Autodesk Fusion 360 part; units mm, degrees
(part 2 of 2)
sketch "Sketch2" plane through (77.4, 0, 0) normal (1, 0, 0) x (0, 1, 0)
  line L0 (0, 36.6134) -> (0, 2)
  line L1 (0, 2) -> (150, 2)
  line L2 (150, 2) -> (150, 36.6134)
  line L3 (150, 36.6134) -> (0, 36.6134)
  line L4 (0, 44) -> (0, 2)
  line L5 (150, 44) -> (0, 44)
  line L6 (150, 11) -> (0, 11)
  line L7 (150, 7) -> (0, 7)
  line L8 (150, 2) -> (150, 44)
  line L9 (0, 2) -> (150, 2)
  line L10 (150, 36) -> (0, 36)
  line L11 (0, 37) -> (150, 37)
  line L12 (150, 29) -> (150, 28)
  line L13 (0, 10) -> (150, 10)
  line L14 (0, 9) -> (0, 10)
  line L15 (150, 38) -> (0, 38)
  line L16 (150, 8) -> (150, 7)
  line L17 (0, 32) -> (0, 33)
  line L18 (150, 35) -> (150, 34)
  line L19 (150, 30) -> (0, 30)
  line L20 (0, 39) -> (150, 39)
  line L21 (150, 9) -> (0, 9)
  line L22 (0, 6) -> (150, 6)
  line L23 (0, 38) -> (0, 39)
  line L24 (0, 28) -> (0, 29)
  line L25 (0, 36) -> (0, 37)
  line L26 (0, 11) -> (0, 12)
  line L27 (0, 29) -> (150, 29)
  line L28 (150, 12) -> (150, 11)
  line L29 (0, 31) -> (150, 31)
  line L30 (150, 5) -> (0, 5)
  line L31 (0, 33) -> (150, 33)
  line L32 (150, 31) -> (150, 30)
  line L33 (0, 35) -> (150, 35)
  line L34 (150, 6) -> (150, 5)
  line L35 (150, 10) -> (150, 9)
  line L36 (150, 28) -> (0, 28)
  line L37 (0, 12) -> (150, 12)
  line L38 (0, 8) -> (150, 8)
  line L39 (150, 37) -> (150, 36)
  line L40 (0, 7) -> (0, 8)
  line L41 (0, 30) -> (0, 31)
  line L42 (0, 34) -> (0, 35)
  line L43 (150, 32) -> (0, 32)
  line L44 (0, 5) -> (0, 6)
  line L45 (150, 39) -> (150, 38)
  line L46 (150, 33) -> (150, 32)
  line L47 (150, 34) -> (0, 34)
  point P0 (150, 0)
  dimension "d78" = 150
  dimension "d79" = 1
  dimension "d80" = 150
  dimension "d81" = 1
  dimension "d82" = 150
  dimension "d83" = 1
  dimension "d84" = 150
  dimension "d85" = 1
  dimension "d86" = 150
  dimension "d87" = 1
  dimension "d88" = 150
  dimension "d89" = 1
  dimension "d90" = 1
  dimension "d91" = 1
  dimension "d92" = 1
  dimension "d93" = 1
  dimension "d94" = 1
  dimension "d96" = 5
  dimension "d97" = 150
  dimension "d98" = 1
  dimension "d99" = 150
  dimension "d100" = 1
  dimension "d101" = 150
  dimension "d102" = 1
  dimension "d103" = 150
  dimension "d104" = 1
  dimension "d105" = 1
  dimension "d106" = 1
  dimension "d107" = 1
  dimension "d108" = 3
  constraint horizontal L20
  constraint vertical L45
  constraint horizontal L15
  constraint vertical L23
  constraint coincident L20.start L4
  constraint horizontal L11
  constraint vertical L39
  constraint horizontal L10
  constraint vertical L25
  constraint coincident L11.start L4
  constraint horizontal L33
  constraint vertical L18
  constraint horizontal L47
  constraint vertical L42
  constraint coincident L33.start L4
  constraint horizontal L29
  constraint vertical L32
  constraint horizontal L19
  constraint vertical L41
  constraint horizontal L31
  constraint vertical L46
  constraint horizontal L43
  constraint vertical L17
  constraint coincident L17.end L4
  constraint horizontal L27
  constraint vertical L12
  constraint horizontal L36
  constraint vertical L24
  constraint coincident L24.end L4
  constraint horizontal L13
  constraint vertical L35
  constraint horizontal L21
  constraint vertical L14
  constraint coincident L13.start L4
  constraint horizontal L38
  constraint vertical L16
  constraint horizontal L7
  constraint vertical L40
  constraint coincident L38.start L4
  constraint horizontal L22
  constraint vertical L34
  constraint horizontal L30
  constraint vertical L44
  constraint coincident L22.start L4
  constraint horizontal L37
  constraint vertical L28
  constraint horizontal L6
  constraint vertical L26
  constraint coincident L26.end L4
  measures "d78" distance of L20.start L20.end
  measures "d79" distance of L20.start L15.end
  measures "d80" distance of L11.end L11.start
  measures "d81" distance of L10.end L11.start
  measures "d82" distance of L33.start L18.start
  measures "d83" distance of L42.start L33.start
  measures "d84" distance of L29.end L29.start
  measures "d85" distance of L19.end L29.start
  measures "d86" distance of L17.end L31.end
  measures "d87" distance of L17.start L17.end
  measures "d88" distance of L12.start L24.end
  measures "d89" distance of L24.start L24.end
  measures "d90" distance of L11 L15
  measures "d91" distance of L10 L33
  measures "d92" distance of L31 L47
  measures "d93" distance of L19 L27
  measures "d94" distance of L29 L43
  measures "d96" distance of L5 L20
  measures "d97" distance of L13.start L13.end
  measures "d98" distance of L13.start L14.start
  measures "d99" distance of L38.start L16.start
  measures "d100" distance of L38.start L7.end
  measures "d101" distance of L22.start L22.end
  measures "d102" distance of L30.end L22.start
  measures "d103" distance of L26.end L28.start
  measures "d104" distance of L26.end L6.end
  measures "d105" distance of L7 L22
  measures "d106" distance of L21 L38
  measures "d107" distance of L6 L13
  measures "d108" distance of L9 L30
extrude "Extrude2" cut sketch "Sketch2" against normal blind 1 contours L0 L2 L4 L8 L18 L33 L42 L47 | L0 L2 L4 L8 L17 L31 L43 L46 | L0 L2 L4 L8 L19 L29 L32 L41 | L0 L2 L4 L8 L12 L24 L27 L36 | L0 L2 L4 L6 L8 L26 L28 L37 | L0 L2 L4 L8 L13 L14 L21 L35 | L0 L2 L4 L7 L8 L16 L38 L40 | L0 L2 L4 L8 L22 L30 L34 L44
sketch "Sketch3" plane through (0, 0, 0) normal (-1, 0, 0) x (0, -1, 0)
  line L0 (0, 2) -> (0, 36.6134)
  line L1 (0, 36.6134) -> (-150, 36.6134)
  line L2 (-150, 36.6134) -> (-150, 2)
  line L3 (-150, 2) -> (0, 2)
  line L4 (-150, 10) -> (-150, 11)
  line L5 (-150, 33) -> (-150, 34)
  line L6 (0, 4) -> (0, 5)
  line L7 (0, 6) -> (0, 7)
  line L8 (0, 8) -> (0, 9)
  line L9 (0, 11) -> (0, 10)
  line L10 (-150, 44) -> (-150, 2)
  line L11 (-150, 30) -> (0, 30)
  line L12 (0, 28) -> (0, 27)
  line L13 (-150, 38) -> (0, 38)
  line L14 (0, 29) -> (-150, 29)
  line L15 (-150, 7) -> (-150, 6)
  line L16 (0, 5) -> (-150, 5)
  line L17 (-150, 34) -> (0, 34)
  line L18 (-150, 37) -> (-150, 38)
  line L19 (-150, 4) -> (0, 4)
  line L20 (0, 37) -> (-150, 37)
  line L21 (-150, 8) -> (0, 8)
  line L22 (0, 33) -> (-150, 33)
  line L23 (-150, 6) -> (0, 6)
  line L24 (0, 7) -> (-150, 7)
  line L25 (-150, 5) -> (-150, 4)
  line L26 (0, 10) -> (-150, 10)
  line L27 (0, 9) -> (-150, 9)
  line L28 (-150, 27) -> (-150, 28)
  line L29 (-150, 11) -> (0, 11)
  line L30 (-150, 29) -> (-150, 30)
  line L31 (-150, 9) -> (-150, 8)
  line L32 (0, 27) -> (-150, 27)
  line L33 (-150, 28) -> (0, 28)
  line L34 (0, 34) -> (0, 33)
  line L35 (0, 31) -> (-150, 31)
  line L36 (0, 32) -> (0, 31)
  line L37 (0, 36) -> (0, 35)
  line L38 (-150, 32) -> (0, 32)
  line L39 (-150, 36) -> (0, 36)
  line L40 (0, 2) -> (0, 44)
  line L41 (0, 44) -> (-150, 44)
  line L42 (-150, 2) -> (0, 2)
  line L43 (0, 38) -> (0, 37)
  line L44 (-150, 31) -> (-150, 32)
  line L45 (-150, 35) -> (-150, 36)
  line L46 (0, 30) -> (0, 29)
  line L47 (0, 35) -> (-150, 35)
  point P0 (-150, 0)
  dimension "d111" = 150
  dimension "d112" = 1
  dimension "d113" = 150
  dimension "d114" = 1
  dimension "d115" = 150
  dimension "d116" = 1
  dimension "d117" = 150
  dimension "d118" = 1
  dimension "d119" = 150
  dimension "d120" = 1
  dimension "d121" = 150
  dimension "d122" = 1
  dimension "d123" = 150
  dimension "d124" = 1
  dimension "d125" = 150
  dimension "d126" = 1
  dimension "d127" = 150
  dimension "d128" = 1
  dimension "d129" = 150
  dimension "d130" = 1
  constraint horizontal L13
  constraint vertical L43
  constraint horizontal L20
  constraint vertical L18
  constraint coincident L13.start L10
  constraint horizontal L39
  constraint vertical L37
  constraint horizontal L47
  constraint vertical L45
  constraint coincident L39.start L10
  constraint horizontal L17
  constraint vertical L34
  constraint horizontal L22
  constraint vertical L5
  constraint coincident L5.end L10
  constraint horizontal L38
  constraint vertical L36
  constraint horizontal L35
  constraint vertical L44
  constraint coincident L38.start L10
  constraint horizontal L11
  constraint vertical L46
  constraint horizontal L14
  constraint vertical L30
  constraint coincident L11.start L10
  constraint horizontal L33
  constraint vertical L12
  constraint horizontal L32
  constraint vertical L28
  constraint coincident L28.end L10
  constraint horizontal L19
  constraint vertical L6
  constraint horizontal L16
  constraint vertical L25
  constraint coincident L19.start L10
  constraint horizontal L23
  constraint vertical L7
  constraint horizontal L24
  constraint vertical L15
  constraint coincident L15.end L10
  constraint horizontal L21
  constraint vertical L8
  constraint horizontal L27
  constraint vertical L31
  constraint coincident L21.start L10
  constraint horizontal L29
  constraint vertical L9
  constraint horizontal L26
  constraint vertical L4
  constraint coincident L4.end L10
  measures "d111" distance of L13.end L13.start
  measures "d112" distance of L18.start L13.start
  measures "d113" distance of L37.start L39.start
  measures "d114" distance of L39.start L45.start
  measures "d115" distance of L17.end L5.end
  measures "d116" distance of L5.start L5.end
  measures "d117" distance of L38.start L36.start
  measures "d118" distance of L35.end L38.start
  measures "d119" distance of L11.start L11.end
  measures "d120" distance of L11.start L14.end
  measures "d121" distance of L28.end L12.start
  measures "d122" distance of L28.end L28.start
  measures "d123" distance of L19.start L6.start
  measures "d124" distance of L16.end L19.start
  measures "d125" distance of L15.end L7.start
  measures "d126" distance of L15.start L15.end
  measures "d127" distance of L8.start L21.start
  measures "d128" distance of L21.start L27.end
  measures "d129" distance of L4.end L9.start
  measures "d130" distance of L4.end L4.start
extrude "Extrude3" cut sketch "Sketch3" against normal blind 1 contours L0 L2 L6 L10 L16 L19 L25 L40 | L0 L2 L7 L10 L15 L23 L24 L40 | L0 L2 L8 L10 L21 L27 L31 L40 | L0 L2 L4 L9 L10 L26 L29 L40 | L0 L2 L10 L12 L28 L32 L33 L40 | L0 L2 L10 L11 L14 L30 L40 L46 | L0 L2 L10 L35 L36 L38 L40 L44 | L0 L2 L5 L10 L17 L22 L34 L40 | L0 L2 L10 L37 L39 L40 L45 L47

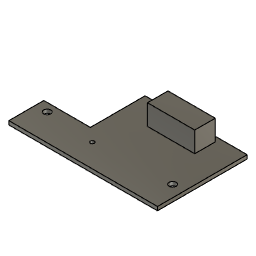
design "InputBoard"
Autodesk Fusion 360 part; units mm, degrees
sketch "Sketch1" plane through (0, 0, 0) normal (0, 0, 1) x (1, 0, 0)
  line L0 (0, 0) -> (63.8, 0)
  line L1 (63.8, 0) -> (63.8, 38.5)
  line L2 (63.8, 38.5) -> (0, 38.5)
  line L3 (0, 38.5) -> (0, 0)
  line L4 (0, 15) -> (20, 15)
  line L5 (20, 15) -> (20, 38.5)
  line L6 (63.8, 38.5) -> (43.8, 38.5)
  line L7 (43.8, 38.5) -> (52.6, 38.5)
  line L8 (52.6, 38.5) -> (52.6, 0)
  line L9 (52.6, 0) -> (43.8, 0)
  line L10 (43.8, 0) -> (43.8, 38.5)
  dimension "d1" = 63.8
  dimension "d2" = 38.5
  dimension "d3" = 20
  dimension "d4" = 15
  dimension "d5" = 20
  dimension "d6" = 8.8
  dimension "d7" = 38.5
  constraint horizontal L0
  constraint vertical L1
  constraint horizontal L2
  constraint vertical L3
  constraint coincident L0.start L3.end
  constraint coincident L3 L4.start
  constraint perpendicular L3 L4
  constraint coincident L2 L5.end
  constraint perpendicular L2 L5
  constraint perpendicular L1 L6
  constraint horizontal L7
  constraint vertical L8
  constraint horizontal L9
  constraint vertical L10
  measures "d1" distance of L0.start L0.end
  measures "d2" distance of L0.start L2.end
  measures "d3" distance of L4.start L4.end
  measures "d4" distance of L0 L4
  measures "d5" distance of L1.end L6.end
  measures "d6" distance of L6.end L7.end
  measures "d7" distance of L6.end L9.end
extrude "Extrude2" add sketch "Sketch1" along normal blind 1.6 contours L0 L2 L3 L4 L5 L10 | L0 L2 L6 L7 L8 L9 L10 | L0 L1 L2 L6 L8
sketch "Sketch4" plane through (0, 0, 1.6) normal (0, 0, 1) x (-1, 0, 0)
  line L0 (-63.8, 0) -> (-63.8, -38.5)
  line L1 (-63.8, -38.5) -> (-20, -38.5)
  line L2 (-20, -38.5) -> (-20, -15)
  line L3 (-20, -15) -> (0, -15)
  line L4 (0, -15) -> (0, 0)
  line L5 (0, 0) -> (-63.8, 0)
  circle A0 centre (-5, -11.5) radius 1.5
  circle A1 centre (-58.8, -11.5) radius 1.5
  dimension "d23" = 3
  dimension "d24" = 11.5
  dimension "d25" = 5
  dimension "d28" = 3
  dimension "d39" = 58.8
  constraint horizontal A0.centre A1.centre
  measures "d23" diameter of A0
  measures "d24" distance of L5 A0.centre
  measures "d25" distance of L4 A0.centre
  measures "d28" diameter of A1
  measures "d39" distance of L4 A1.centre
extrude "Extrude5" cut sketch "Sketch4" against normal blind 1.6 contours A0
hole "Hole1" at (58.8, 11.5, 1.6) direction (0, 0, -1) diameter 3 depth 5 tip angle 180
sketch "Sketch5" plane through (0, 0, 1.6) normal (0, 0, 1) x (1, 0, 0)
  circle A0 centre (25.907, 9.929) radius 0.85
  line L0 (0, 0) -> (63.8, 0)
  line L1 (0, 15) -> (0, 0)
  dimension "d34" = 1.7
  dimension "d35" = 9.929
  dimension "d36" = 25.907
  measures "d34" diameter of A0
  measures "d35" distance of A0.centre L0
  measures "d36" distance of A0.centre L1
extrude "Extrude6" cut sketch "Sketch5" against normal blind 1.6
sketch "Sketch6" plane through (0, 0, 1.6) normal (0, 0, 1) x (-1, 0, 0)
  circle A0 centre (-25.907, -9.929) radius 0.85
  circle A1 centre (-58.8, -11.5) radius 1.5
  circle A2 centre (-5, -11.5) radius 1.5
  line L0 (-63.8, 0) -> (-63.8, -38.5)
  line L1 (-63.8, -38.5) -> (-20, -38.5)
  line L2 (-20, -38.5) -> (-20, -15)
  line L3 (-20, -15) -> (0, -15)
  line L4 (0, -15) -> (0, 0)
  line L5 (0, 0) -> (-63.8, 0)
  line L6 (-52.187, -27.604) -> (-31.887, -27.604)
  line L7 (-31.887, -27.604) -> (-31.887, -36.404)
  line L8 (-31.887, -36.404) -> (-52.187, -36.404)
  line L9 (-52.187, -36.404) -> (-52.187, -27.604)
  line L10 (-52.187, -27.604) -> (-31.887, -36.404) construction
  line L11 (-31.887, -27.604) -> (-52.187, -36.404) construction
  point P0 (-42.037, -32.004)
  dimension "d40" = 20.3
  dimension "d41" = 8.8
  dimension "d42" = 42.037
  dimension "d43" = 32.004
  constraint horizontal L6
  constraint perpendicular L6 L7
  constraint parallel L6 L8
  constraint parallel L7 L9
  constraint coincident L10 P0
  constraint coincident L11 P0
  measures "d40" distance of L7.end L8.end
  measures "d41" distance of L6.end L7.end
  measures "d42" horizontal distance of L4.end P0
  measures "d43" vertical distance of L4.end P0
extrude "Extrude7" add sketch "Sketch6" along normal blind 8.8 contours L6 L7 L8 L9

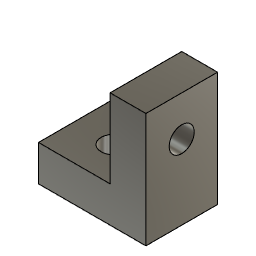
design "Output_Top_Stand"
Autodesk Fusion 360 part; units mm, degrees
sketch "Sketch1" plane through (0, 0, 0) normal (0, 0, 1) x (1, 0, 0)
  line L0 (0, 0) -> (15, 0)
  line L1 (15, 0) -> (15, 10)
  line L2 (15, 10) -> (0, 10)
  line L3 (0, 10) -> (0, 0)
  line L4 (15, 5) -> (5.5, 5)
  circle A0 centre (5.5, 5) radius 1.75
  dimension "d1" = 15
  dimension "d2" = 10
  dimension "d27" = 9.5
  dimension "d28" = 3.5
  constraint horizontal L0
  constraint vertical L1
  constraint horizontal L2
  constraint vertical L3
  constraint coincident L0.start L3.end
  constraint midpoint L1 L4.start
  constraint perpendicular L1 L4
  constraint coincident L4.end A0.centre
  measures "d1" distance of L0.start L0.end
  measures "d2" distance of L0.start L2.end
  measures "d27" distance of L4.start L4.end
  measures "d28" diameter of A0
extrude "Extrude1" add sketch "Sketch1" along normal blind 5 contours L0 L1 L2 L3 | A0
extrude "Extrude4" cut sketch "Sketch1" along normal blind 5 contours A0
sketch "Sketch5" plane through (0, 0, 0) normal (0, 0, -1) x (1, 0, 0)
  circle A0 centre (5.5, -5) radius 1.75
  line L0 (0, 0) -> (0, -10)
  line L1 (0, -10) -> (15, -10)
  line L2 (15, -10) -> (15, 0)
  line L3 (15, 0) -> (0, 0)
  line L4 (15, 0) -> (10, 0)
  line L5 (10, 0) -> (10, -10)
  line L6 (10, -10) -> (15, -10)
  line L7 (15, -10) -> (15, 0)
  dimension "d31" = 5
  dimension "d32" = 10
  constraint horizontal L4
  constraint vertical L5
  constraint horizontal L6
  constraint vertical L7
  constraint coincident L2.end L3.start
  measures "d31" distance of L2.end L4.end
  measures "d32" distance of L2.end L1.end
extrude "Extrude5" add sketch "Sketch5" against normal blind 16 contours L1 L2 L3 L4 L5 L6 L7
sketch "Sketch6" plane through (15, 0, 0) normal (1, 0, 0) x (0, 1, 0)
  line L0 (0, 0) -> (10, 0)
  line L1 (10, 0) -> (10, 16)
  line L2 (10, 16) -> (0, 16)
  line L3 (0, 16) -> (0, 0)
  line L4 (5, 0) -> (5, 10.4)
  circle A0 centre (5, 10.4) radius 1.75
  dimension "d35" = 10.4
  dimension "d36" = 3.5
  constraint midpoint L0 L4.start
  constraint perpendicular L0 L4
  constraint coincident L4.end A0.centre
  measures "d35" distance of L4.start L4.end
  measures "d36" diameter of A0
extrude "Extrude6" cut sketch "Sketch6" against normal blind 5 contours A0
